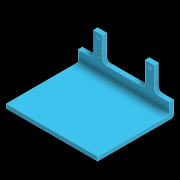
# Autodesk Inventor part: 零件12
Saved by Autodesk Inventor 2020 (Build 240168000, 168)
## iProperties
Created: 2021-04-08
Part Number: 零件12
Material: 一般
Document SubType Name: Modeling
Designer: 88690
Density: 1 g/cm^3
Appearance: 青綠色
Author: 88690
Autodesk Inventor part; units mm, degrees
ref_plane "YZ Plane" through (0, 0, 0) normal (1, 0, 0) x (0, 1, 0)
ref_plane "XZ Plane" through (0, 0, 0) normal (0, 1, 0) x (-1, 0, 0)
ref_plane "XY Plane" through (0, 0, 0) normal (0, 0, 1) x (1, 0, 0)
sketch "草圖1" plane through (0, 0, 0) normal (0, 0, 1) x (1, 0, 0)
  line L0 (0, 0) -> (0, 117.5667) construction
  line L1 (-139.2449, 0) -> (139.2449, 0) construction
  line L2 (-110, 88) -> (-77, 88)
  line L3 (-77, 88) -> (-77, 0)
  line L4 (-77, 0) -> (-110, 0)
  line L5 (-110, 0) -> (-110, 88)
  line L6 (77, 88) -> (110, 88)
  line L7 (110, 88) -> (110, 0)
  line L8 (110, 0) -> (77, 0)
  line L9 (77, 0) -> (77, 88)
  line L10 (-110, 0) -> (-77, 0)
  line L11 (-77, 0) -> (-77, -55)
  line L12 (-77, -55) -> (-110, -55)
  line L13 (-110, -55) -> (-110, 0)
  line L14 (77, 0) -> (110, 0)
  line L15 (110, 0) -> (110, -55)
  line L16 (110, -55) -> (77, -55)
  line L17 (77, -55) -> (77, 0)
  dimension "d0" = 33
  dimension "d1" = 33
  dimension "d2" = 220
  dimension "d3" = 110
  dimension "d4" = 88
  dimension "d5" = 88
  dimension "d6" = 55
  dimension "d7" = 55
  constraints: 36 end point, 8 parallel, 5 horizontal, 4 collinear, 4 perpendicular, 1 midpoint, 1 vertical
  measures "d0" distance of L2.start L2.end
  measures "d1" distance of L6.start L6.end
  measures "d2" distance between parallel lines of L5 L7
  measures "d3" distance between parallel lines of L7 L0
  measures "d4" distance of L6.end L7.end
  measures "d5" distance of L4.end L2.start
  measures "d6" distance of L12.end L4.end
  measures "d7" distance of L14.end L15.end
extrude "擠出1" add sketch "草圖1" along normal blind 15
sketch "草圖2" plane through (0, 0, 15) normal (0, 0, 1) x (1, 0, 0)
  line L0 (-77, -55) -> (-110, -55) construction
  line L1 (-110, -55) -> (-110, 88) construction
  line L2 (-110, 88) -> (-77, 88) construction
  line L3 (-77, 88) -> (-77, -55) construction
  line L4 (77, 88) -> (110, 88) construction
  line L5 (110, 88) -> (110, -55) construction
  line L6 (110, -55) -> (77, -55) construction
  line L7 (77, -55) -> (77, 88) construction
  line L8 (-110, -55) -> (110, -55)
  line L9 (110, -55) -> (110, -40)
  line L10 (110, -40) -> (-110, -40)
  line L11 (-110, -40) -> (-110, -55)
  point P0 (0, 0)
  dimension "d10" = 15
  constraints: 8 end point, 2 parallel, 1 horizontal, 1 perpendicular, 1 point on line
  measures "d10" distance between parallel lines of L8 L10
extrude "擠出2" add sketch "草圖2" along normal blind 260
sketch "草圖3" plane through (0, 0, 15) normal (0, 0, 1) x (1, 0, 0)
  circle A0 centre (-93.5, 71.5) radius 6
  circle A1 centre (-93.5, 16.5) radius 6
  circle A2 centre (93.5, 71.5) radius 6
  circle A3 centre (93.5, 16.5) radius 6
  line L0 (110, 88) -> (77, 88) construction
  line L1 (-77, 88) -> (-110, 88) construction
  line L2 (-93.5, 88) -> (-93.5, -40) construction
  line L3 (-110, -40) -> (-77, -40) construction
  line L4 (93.5, 88) -> (93.5, -40) construction
  line L5 (110, -40) -> (-110, -40) construction
  point P0 (0, 0)
  dimension "d13" = 55
  dimension "d14" = 12
  dimension "d15" = 12
  dimension "d16" = 12
  dimension "d17" = 12
  dimension "d18" = 55
  dimension "d19" = 16.5
  dimension "d20" = 16.5
  constraints: 5 point on line, 4 centre point, 4 end point, 3 midpoint, 1 vertical
  measures "d13" distance of A2.centre A3.centre
  measures "d14" diameter of A2
  measures "d15" diameter of A3
  measures "d16" diameter of A0
  measures "d17" diameter of A1
  measures "d18" distance of A0.centre A1.centre
  measures "d19" distance from line of L0 A2.centre
  measures "d20" distance from line of L1 A0.centre
extrude "擠出3" cut sketch "草圖3" against normal blind 200
sketch "草圖4" plane through (-110, -55, 0) normal (0, -1, 0) x (1, 0, 0)
  line L0 (187, 15) -> (33, 15) construction
  line L1 (33, 15) -> (33, 0) construction
  line L2 (33, 0) -> (0, 0) construction
  line L3 (0, 0) -> (0, 275) construction
  line L4 (0, 275) -> (220, 275) construction
  line L5 (220, 275) -> (220, 0) construction
  line L6 (220, 0) -> (187, 0) construction
  line L7 (187, 0) -> (187, 15) construction
  line L8 (-55, 275) -> (275, 275)
  line L9 (275, 275) -> (275, 15)
  line L10 (275, 15) -> (-55, 15)
  line L11 (-55, 15) -> (-55, 275)
  point P0 (110, 0)
  point P1 (110, 275)
  point P2 (110, 15)
  dimension "d23" = 55
  constraints: 8 end point, 4 midpoint, 2 parallel, 1 horizontal, 1 perpendicular
  measures "d23" distance between parallel lines of L9 L5
extrude "擠出4" add sketch "草圖4" against normal blind 15
sketch "草圖5" plane through (0, 0, 15) normal (0, 0, -1) x (-1, 0, 0)
  circle A0 centre (-93.5, 71.5) radius 6 construction
  circle A1 centre (93.5, 71.5) radius 6 construction
  circle A2 centre (-93.5, 16.5) radius 6 construction
  circle A3 centre (93.5, 16.5) radius 6 construction
  line L0 (-110, 88) -> (-77, 88) construction
  line L1 (-77, 88) -> (-77, -40) construction
  line L2 (-77, -40) -> (77, -40) construction
  line L3 (77, -55) -> (77, -40) construction
  line L4 (77, -55) -> (-77, -55) construction
  line L5 (-77, -55) -> (-110, -55) construction
  line L6 (-110, -55) -> (-110, -40) construction
  line L7 (-110, -40) -> (-77, -40) construction
  line L8 (-110, -40) -> (-110, 88) construction
  line L9 (-165, -40) -> (-110, -40) construction
  line L10 (-165, -55) -> (-165, -40) construction
  line L11 (-110, -55) -> (-165, -55) construction
  line L12 (-77, -40) -> (-77, -55) construction
  line L13 (77, -40) -> (110, -40) construction
  line L14 (110, -40) -> (110, -55) construction
  line L15 (165, -55) -> (110, -55) construction
  line L16 (165, -40) -> (165, -55) construction
  line L17 (110, -40) -> (165, -40) construction
  line L18 (110, 88) -> (110, -40) construction
  line L19 (77, 88) -> (110, 88) construction
  line L20 (77, -40) -> (77, 88) construction
  line L21 (110, -55) -> (77, -55) construction
  line L22 (-165, -55) -> (165, -55)
  line L23 (165, -55) -> (165, 0)
  line L24 (165, 0) -> (-165, 0)
  line L25 (-165, 0) -> (-165, -55)
  line L26 (165, -55) -> (165, -40) projected
  point P0 (0, 0)
  dimension "d26" = 40
  constraints: 8 end point, 2 parallel, 1 collinear, 1 horizontal, 1 perpendicular
  measures "d26" distance between parallel lines of L24 L17
extrude "擠出5" add sketch "草圖5" along normal blind 15
fillet "圓角1" radius 10 1 edges at (0, -55, 0)
fillet "圓角2" radius 5 1 edges at (0, -40, 15)
fillet "圓角3" radius 15 4 edges at (-77, 0, 7.5) (-110, 0, 7.5) (77, 0, 7.5) (110, 0, 7.5)
equation "\"d3\" = 0.5 * d2"
equation "\"d15\" = d14"
equation "\"d16\" = d14"
equation "\"d17\" = d14"
equation "\"d18\" = d13"
equation "\"d20\" = d19"
